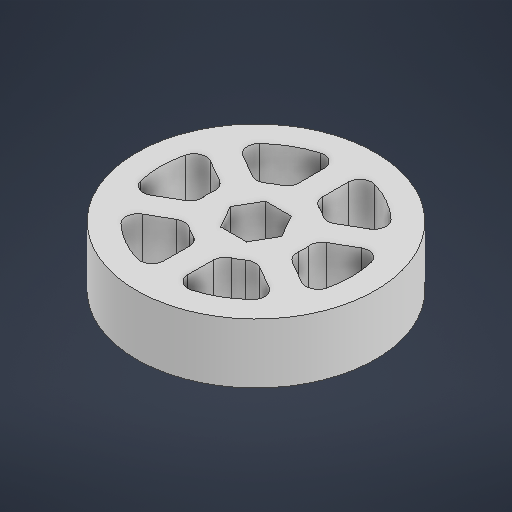
# Autodesk Inventor part: 2in mould
Saved by Autodesk Inventor 2025.2 (Build 292293000, 293)
## iProperties
Created: 2026-01-14
Part Number: 2in mould
Material: Generic
Document SubType Name: Modeling
Designer: cloudy
Density: 1 g/cm^3
Appearance: Default
Author: cloudy
Autodesk Inventor part; units mm, degrees
ref_plane "YZ Plane" through (0, 0, 0) normal (1, 0, 0) x (0, 1, 0)
ref_plane "XZ Plane" through (0, 0, 0) normal (0, 1, 0) x (-1, 0, 0)
ref_plane "XY Plane" through (0, 0, 0) normal (0, 0, 1) x (1, 0, 0)
sketch "Sketch1" plane through (0, 0, 0) normal (0, 1, 0) x (-1, 0, 0)
  circle A0 centre (0, 0) radius 25.4
  line L0 (-2.7424, 4.75) -> (2.7424, 4.75)
  line L1 (2.7424, 4.75) -> (5.4848, 0)
  line L2 (5.4848, 0) -> (2.7424, -4.75)
  line L3 (2.7424, -4.75) -> (-2.7424, -4.75)
  line L4 (-2.7424, -4.75) -> (-5.4848, 0)
  line L5 (-5.4848, 0) -> (-2.7424, 4.75)
  line L6 (2.54, -9.8374) -> (2.54, -20.1606)
  line L7 (-2.54, -9.8374) -> (-2.54, -20.1606)
  line L8 (0, -11.1125) -> (0, -22.225) construction
  line L9 (9.7894, -2.719) -> (18.7296, -7.8806)
  line L10 (7.2494, -7.1184) -> (16.1896, -12.28)
  line L11 (7.2494, 7.1184) -> (16.1896, 12.28)
  line L12 (9.7894, 2.719) -> (18.7296, 7.8806)
  line L13 (-2.54, 9.8374) -> (-2.54, 20.1606)
  line L14 (2.54, 9.8374) -> (2.54, 20.1606)
  line L15 (-9.7894, 2.719) -> (-18.7296, 7.8806)
  line L16 (-7.2494, 7.1184) -> (-16.1896, 12.28)
  line L17 (-7.2494, -7.1184) -> (-16.1896, -12.28)
  line L18 (-9.7894, -2.719) -> (-18.7296, -7.8806)
  arc A1 (9.7894, -2.719) -> (9.7894, 2.719) centre (0, 0) ccw
  arc A2 (7.2494, 7.1184) -> (2.54, 9.8374) centre (0, 0) ccw
  arc A3 (-2.54, 9.8374) -> (-7.2494, 7.1184) centre (0, 0) ccw
  arc A4 (-9.7894, 2.719) -> (-9.7894, -2.719) centre (0, 0) ccw
  arc A5 (-16.1896, -12.28) -> (-2.54, -20.1606) centre (0, 0) ccw
  arc A6 (2.54, -20.1606) -> (16.1896, -12.28) centre (0, 0) ccw
  arc A7 (18.7296, -7.8806) -> (18.7296, 7.8806) centre (0, 0) ccw
  arc A8 (16.1896, 12.28) -> (2.54, 20.1606) centre (0, 0) ccw
  arc A9 (-2.54, 20.1606) -> (-16.1896, 12.28) centre (0, 0) ccw
  arc A10 (-18.7296, 7.8806) -> (-18.7296, -7.8806) centre (0, 0) ccw
  arc A11 (-7.2494, -7.1184) -> (-2.54, -9.8374) centre (0, 0) ccw
  arc A12 (2.54, -9.8374) -> (7.2494, -7.1184) centre (0, 0) ccw
  dimension "d1" = 9.5
  dimension "d4" = 5.08
  dimension "d7" = 360
  dimension "d9" = 20.32
  dimension "d10" = 10.16
  dimension "d11" = 25.4
  constraints: 38 end point, 24 point on circle, 13 centre point, 4 coincident, 3 vertical, 1 horizontal, 1 point on line, 51 other
  measures "d1" distance between parallel lines of L0 L3
  measures "d4" distance between parallel lines of L6 L7
  measures "d9" radius of A5
  measures "d10" radius of A11
  measures "d11" radius of A0
extrude "Extrusion1" add sketch "Sketch1" along normal blind 12.7
fillet "Fillet1" radius 2.54 4 edges at (16.1896, 6.35, 12.28) (7.2494, 6.35, 7.1184) (2.54, 6.35, 9.8374) (2.54, 6.35, 20.1606)
pattern_circular "Circular Pattern1" count 6 over 360 about axis through (0, 0, 0) along (0, 1, 0) of "Fillet1"
body "Solid1"
